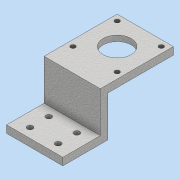
# Autodesk Inventor part: Uchwyt silnika krokowego osi Y
Saved by Autodesk Inventor 2018 (Build 220112000, 112)
## iProperties
Created: 2019-01-25
Part Number: Uchwyt silnika krokowego osi Y
Material: Ogólny
Document SubType Name: Modeling
Designer: Dawid
Density: 1 g/cm^3
Appearance: Aluminium odlewane
Author: Dawid
Autodesk Inventor part; units mm, degrees
ref_plane "YZ Plane" through (0, 0, 0) normal (1, 0, 0) x (0, 1, 0)
ref_plane "XZ Plane" through (0, 0, 0) normal (0, 1, 0) x (-1, 0, 0)
ref_plane "XY Plane" through (0, 0, 0) normal (0, 0, 1) x (1, 0, 0)
sketch "Szkic1" plane through (0, 0, 0) normal (0, 0, 1) x (1, 0, 0)
  line L0 (-30, -35) -> (30, -35)
  line L1 (30, -35) -> (30, 35)
  line L2 (30, 35) -> (-30, 35)
  line L3 (-30, 35) -> (-30, -35)
  line L4 (-30, -35) -> (30, 35) construction
  line L5 (30, -35) -> (-30, 35) construction
  point P0 (0, 0)
  dimension "d0" = 60
  dimension "d1" = 70
  constraints: 12 end point, 2 midpoint, 2 parallel, 1 horizontal, 1 perpendicular
  measures "d0" distance of L2.end L1.end
  measures "d1" distance of L1.end L0.end
extrude "Wyciągnięcie proste1" add sketch "Szkic1" along normal blind 8
sketch "Szkic2" plane through (0, 0, 0) normal (0, 0, -1) x (-1, 0, 0)
  line L0 (30, -35) -> (-30, -35) projected
  line L1 (30, 35) -> (30, -35) projected
  line L2 (-30, 35) -> (30, 35) projected
  line L3 (-30, -35) -> (-30, 35) projected
  line L4 (23.57, 5) -> (23.57, 28.57)
  line L5 (23.57, 28.57) -> (-23.57, 28.57)
  line L6 (-23.57, 28.57) -> (-23.57, -18.57)
  line L7 (-23.57, -18.57) -> (23.57, -18.57)
  line L8 (23.57, -18.57) -> (23.57, 5)
  circle A0 centre (23.57, 28.57) radius 2.5
  circle A1 centre (-23.57, 28.57) radius 2.5
  circle A2 centre (-23.57, -18.57) radius 2.5
  circle A3 centre (23.57, -18.57) radius 2.5
  line L9 (0, 0) -> (0, 5)
  dimension "d6" = 47.14
  dimension "d7" = 47.14
  dimension "d8" = 47.14
  dimension "d9" = 5
  dimension "d10" = 5
  dimension "d11" = 5
  dimension "d12" = 5
  dimension "d15" = 5
  constraints: 12 end point, 4 centre point, 4 coincident, 2 perpendicular, 1 point on line, 1 vertical
  measures "d6" distance of L4.end L5.end
  measures "d7" distance of L5.end L6.end
  measures "d8" distance of L6.end L7.end
  measures "d9" diameter of A0
  measures "d10" diameter of A1
  measures "d11" diameter of A2
  measures "d12" diameter of A3
  measures "d15" distance of L9.start L9.end
extrude "Wyciągnięcie proste3" cut sketch "Szkic2" against normal up to next contours A0 L5 L4 | L4 L5 A0 | A3 L7 L8 | L8 L7 A3 | A1 L6 L5 | L5 L6 A1 | A2 L6 L7 | L7 L6 A2
sketch "Szkic4" plane through (0, 0, 8) normal (0, 0, 1) x (1, 0, 0)
  line L0 (-30, -35) -> (30, -35) projected
  line L1 (30, -35) -> (30, -43)
  line L2 (30, -43) -> (-30, -43)
  line L3 (-30, -43) -> (-30, -35)
  point P0 (0, 0)
  dimension "d18" = 8
  constraints: 6 end point, 2 perpendicular, 1 vertical
  measures "d18" distance of L0.end L1.end
extrude "Wyciągnięcie proste4" add sketch "Szkic4" against normal blind 43.4
sketch "Szkic5" plane through (0, 0, 8) normal (0, 0, 1) x (1, 0, 0)
  circle A0 centre (-23.57, -18.57) radius 2.5 projected
  circle A1 centre (23.57, 28.57) radius 2.5 projected
  circle A2 centre (-23.57, 28.57) radius 2.5 projected
  circle A3 centre (23.57, -18.57) radius 2.5 projected
  line L0 (30, 35) -> (30, -43) projected
  line L1 (30, 35) -> (-30, 35) projected
  line L2 (-30, 35) -> (-30, -43) projected
  line L3 (30, -43) -> (-30, -43) projected
  line L4 (23.57, -18.57) -> (-23.57, 28.57)
  line L5 (-23.57, -18.57) -> (23.57, 28.57)
  circle A4 centre (0, 5) radius 15
  point P0 (0, 0)
  dimension "d21" = 30
  constraints: 4 end point, 1 centre point, 1 midpoint
  measures "d21" diameter of A4
extrude "Wyciągnięcie proste5" cut sketch "Szkic5" against normal up to next contours A4 L5 L4 | L4 L5 A4 | L5 A4 L4 | L4 A4 L5
thread "Gwint1" size "M5x0.8" class "6H" standard "ANSI Metric M Profile" full length
thread "Gwint2" size "M5x0.8" class "6H" standard "ANSI Metric M Profile" full length
thread "Gwint3" size "M5x0.8" class "6H" standard "ANSI Metric M Profile" full length
thread "Gwint4" size "M5x0.8" class "6H" standard "ANSI Metric M Profile" full length
sketch "Szkic8" plane through (-30, -35, 0) normal (0, 1, 0) x (1, 0, 0)
  line L0 (0, 35.4) -> (60, 35.4) projected
  line L1 (0, 35.4) -> (0, 43.4)
  line L2 (0, 43.4) -> (60, 43.4)
  line L3 (60, 43.4) -> (60, 35.4)
  point P0 (30, 0)
  dimension "d46" = 8
  constraints: 6 end point, 2 perpendicular, 1 vertical
  measures "d46" distance of L0.start L1.end
extrude "Wyciągnięcie proste8" add sketch "Szkic8" against normal blind 48
sketch "Szkic9" plane through (30, -35, -43.4) normal (0, 0, -1) x (-1, 0, 0)
  line L0 (0, 0) -> (60, 0) projected
  line L1 (0, 0) -> (0, -48) projected
  line L2 (60, -48) -> (0, -48) projected
  line L3 (60, 0) -> (60, -48) projected
  line L4 (60, -8) -> (60, -48) projected
  line L5 (60, -48) -> (60, -38)
  line L6 (60, -38) -> (0, -38)
  line L7 (60, -38) -> (60, -18)
  line L8 (60, -18) -> (0, -18)
  line L9 (0, -8) -> (0, -48) projected
  line L10 (0, -48) -> (15, -48)
  line L11 (0, -48) -> (60, -48) projected
  line L12 (15, -48) -> (15, -18)
  line L13 (60, -48) -> (45, -48)
  line L14 (45, -48) -> (45, -18)
  circle A0 centre (45, -38) radius 3
  circle A1 centre (15, -38) radius 3
  circle A2 centre (45, -18) radius 3
  circle A3 centre (15, -18) radius 3
  point P0 (30, 35)
  dimension "d49" = 10
  dimension "d50" = 20
  dimension "d51" = 15
  dimension "d52" = 15
  dimension "d53" = 6
  dimension "d54" = 6
  dimension "d55" = 6
  dimension "d56" = 6
  constraints: 16 end point, 12 point on line, 4 centre point, 4 perpendicular, 2 coincident
  measures "d49" distance of L2.start L5.end
  measures "d50" distance of L5.end L7.end
  measures "d51" distance of L1.end L10.end
  measures "d52" distance of L2.start L13.end
  measures "d53" diameter of A0
  measures "d54" diameter of A1
  measures "d55" diameter of A2
  measures "d56" diameter of A3
extrude "Wyciągnięcie proste9" cut sketch "Szkic9" against normal up to next contours A3 L8 | L8 L12 A3 | A2 L14 L8 | L8 A2 | A1 L12 L6 | L6 L12 A1 | L8 A3 L12 | A0 L14 L6 | L6 L14 A0 | L14 A2 L8 | L12 A1 L6 | L6 A1 L12 | L14 A0 L6 | L6 A0 L14
sketch "Szkic10" plane through (0, 0, 0) normal (0, 0, -1) x (-1, 0, 0)
  circle A0 centre (0, 5) radius 15 projected
  circle A1 centre (0, 5) radius 19.5
  point P0 (0, 0)
  dimension "d59" = 39
  constraints: 1 centre point, 1 coincident
  measures "d59" diameter of A1
extrude "Wyciągnięcie proste10" cut sketch "Szkic10" against normal blind 2
